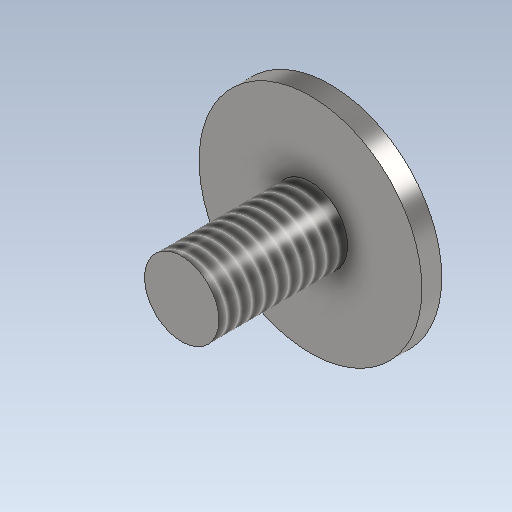
# Autodesk Inventor part: FreeHorn_Screw
Saved by Autodesk Inventor 2020 (Build 240168000, 168)
## iProperties
Created: 2021-08-23
Part Number: FreeHorn_Screw
Material: ステンレス鋼 AISI 304
Document SubType Name: Modeling
Designer: MasatoKubotera
Density: 8 g/cm^3
Appearance: 半つや出し
Description: ネジ
Mass: 0.701203 g
Surface Area: 1.98863 cm^2
Volume: 0.0876504 cm^3
Author: MasatoKubotera
Comments: https://kondo-robot.com/product/02137
Autodesk Inventor part; units mm, degrees
ref_plane "YZ Plane" through (0, 0, 0) normal (1, 0, 0) x (0, 1, 0)
ref_plane "XZ Plane" through (0, 0, 0) normal (0, 1, 0) x (-1, 0, 0)
ref_plane "XY Plane" through (0, 0, 0) normal (0, 0, 1) x (1, 0, 0)
sketch "スケッチ1" plane through (0, 0, 0) normal (0, 0, 1) x (1, 0, 0)
  circle A0 centre (0, 0) radius 4.5
  circle A1 centre (0, 0) radius 1.5
  dimension "d0" = 9
  dimension "d1" = 3
  constraints: 2 centre point, 2 coincident
  measures "d0" diameter of A0
  measures "d1" diameter of A1
extrude "押し出し1" add sketch "スケッチ1" along normal blind 0.8 contours A0 | A1
extrude "押し出し2" add sketch "スケッチ1" along normal blind 6 contours A1
thread "ねじ1" size "M3x0.5" class "6g" standard "ANSI Metric M Profile" full length
